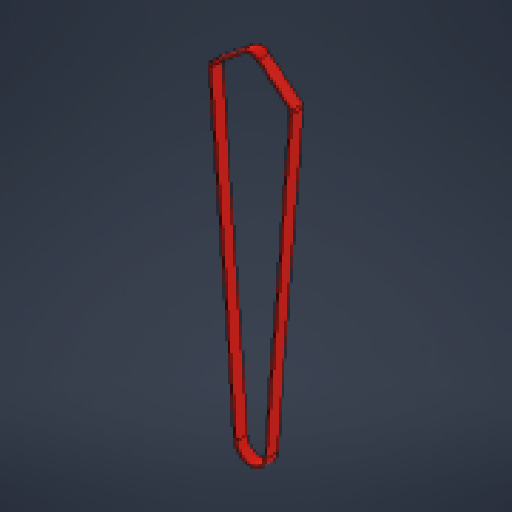
# Autodesk Inventor part: Compression bar band
Saved by Autodesk Inventor 2023.2 (Build 272271030, 271C)
## iProperties
Created: 2023-04-07
Part Number: Compression bar band
Material: Generic
Document SubType Name: Modeling
Designer: Main Account
Density: 1 g/cm^3
Appearance: Default
Author: Main Account
Autodesk Inventor part; units mm, degrees
ref_plane "YZ Plane" through (0, 0, 0) normal (1, 0, 0) x (0, 1, 0)
ref_plane "XZ Plane" through (0, 0, 0) normal (0, 1, 0) x (-1, 0, 0)
ref_plane "XY Plane" through (0, 0, 0) normal (0, 0, 1) x (1, 0, 0)
sketch "Sketch1" plane through (0, 0, 0) normal (0, 0, 1) x (1, 0, 0)
  circle A0 centre (-6, 6) radius 6.35 construction
  arc A1 (-12.3293, 5.4878) -> (0.3289, 5.4825) centre (-6, 6) ccw
  circle A2 centre (-5.9366, 155.7806) radius 4.7625 construction
  arc A3 (-2.9248, 159.4699) -> (-8.9453, 159.4724) centre (-5.9366, 155.7806) ccw
  line L0 (-23.7206, 146.2632) -> (-23.7201, 147.4316) construction
  line L1 (11.8399, 147.4165) -> (11.8394, 146.2481) construction
  line L2 (-8.9453, 159.4724) -> (-23.7201, 147.4316)
  line L3 (0.3289, 5.4825) -> (11.8394, 146.2481)
  line L4 (11.8399, 147.4165) -> (11.8394, 146.2481)
  line L5 (11.8399, 147.4165) -> (-2.9248, 159.4699)
  line L6 (-23.7201, 147.4316) -> (-23.7206, 146.2632)
  line L7 (-23.7206, 146.2632) -> (-12.3293, 5.4878)
  line L8 (12.8393, 146.2071) -> (1.3255, 5.401)
  arc A4 (-13.3261, 5.4072) -> (1.3255, 5.401) centre (-6, 6) ccw
  line L9 (-13.3261, 5.4072) -> (-24.7206, 146.223)
  line L10 (-24.7206, 146.223) -> (-24.7199, 147.9068)
  line L11 (-24.7199, 147.9068) -> (-9.577, 160.2476)
  arc A5 (-2.2924, 160.2445) -> (-9.577, 160.2476) centre (-5.9366, 155.7806) ccw
  line L12 (-2.2924, 160.2445) -> (12.8401, 147.8909)
  line L13 (12.8401, 147.8909) -> (12.8393, 146.2071)
  point P0 (0, 0)
  dimension "d7" = 1
  constraints: 24 end point, 8 point on circle, 4 centre point, 4 tangent, 2 coincident, 2 concentric, 1 collinear, 7 other
  measures "d7" distance between parallel lines of L3 L8
extrude "Extrusion1" add sketch "Sketch1" along normal blind 5
body "Solid1"
